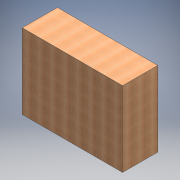
# Autodesk Inventor part: Robot Volume and wall
Saved by Autodesk Inventor 2016 (Build 200138000, 138)
## iProperties
Created: 2017-12-21
Part Number: Robot Volume and wall
Material: Wood (Birch)
Document SubType Name: Modeling
Designer: kornbot
Density: 0.55 g/cm^3
Appearance: Birch - Natural Polished
Author: kornbot
Autodesk Inventor part; units mm, degrees
ref_plane "YZ Plane" through (0, 0, 0) normal (1, 0, 0) x (0, 1, 0)
ref_plane "XZ Plane" through (0, 0, 0) normal (0, 1, 0) x (-1, 0, 0)
ref_plane "XY Plane" through (0, 0, 0) normal (0, 0, 1) x (1, 0, 0)
sketch "Sketch1" plane through (0, 0, 0) normal (0, 0, 1) x (1, 0, 0)
  line L0 (0, 0) -> (0, 700)
  line L1 (0, 0) -> (2000, 0)
  line L2 (0, 700) -> (2000, 700)
  line L3 (2000, 700) -> (2000, 0)
  line L4 (2000, 0) -> (0, 0)
  line L5 (0, 0) -> (0, 700)
  dimension "d0" = 700
  dimension "d1" = 2000
  constraints: 12 end point, 2 horizontal, 2 parallel, 1 perpendicular, 1 vertical
  measures "d0" distance of L0.start L0.end
  measures "d1" distance of L0.start L1.end
extrude "Extrusion1" add sketch "Sketch1" along normal blind 1500
sketch "Sketch2" plane through (0, 700, 0) normal (0, 1, 0) x (1, 0, 0)
  line L0 (1974.1538, -1477.007) -> (20.8481, -1477.007)
  line L1 (20.8481, -1477.007) -> (20.8481, -20.8481)
  line L2 (20.8481, -20.8481) -> (1974.1538, -20.8481)
  line L3 (1974.1538, -20.8481) -> (1974.1538, -1477.007)
  point P0 (0, 0)
  constraints: 8 end point, 2 parallel, 1 horizontal, 1 perpendicular
extrude "Extrusion2" cut sketch "Sketch2" against normal blind 692.25
sketch "Sketch3" plane through (0, 7.75, 0) normal (0, 1, 0) x (1, 0, 0)
  line L0 (1974.1538, -20.8481) -> (1974.1538, -1477.007) projected
  line L1 (20.8481, -20.8481) -> (1974.1538, -20.8481) projected
  line L2 (1974.1538, -1477.007) -> (20.8481, -20.8481)
  line L3 (1974.1538, -1477.007) -> (20.8481, -1477.007) projected
  line L4 (20.8481, -1477.007) -> (1974.1538, -20.8481)
  line L5 (997.5009, -748.9276) -> (997.5009, -1112.664)
  circle A0 centre (997.5009, -1112.664) radius 140.4471
  line L6 (997.5009, -1253.1111) -> (997.5009, -1303.1111)
  circle A1 centre (997.5009, -1303.1111) radius 25
  circle A2 centre (832.5689, -1207.8876) radius 25
  circle A3 centre (832.5689, -1017.4404) radius 25
  circle A4 centre (997.5009, -922.2169) radius 25
  circle A5 centre (1162.433, -1017.4404) radius 25
  circle A6 centre (1162.433, -1207.8876) radius 25
  circle A7 centre (997.5009, -1112.664) radius 226.7645
  circle A8 centre (997.5009, -1112.664) radius 226.7645
  point P0 (0, 0)
  dimension "d9" = 50
  dimension "d11" = 50
  dimension "d14" = 360
  constraints: 8 centre point, 8 end point, 4 coincident, 2 midpoint, 2 vertical, 1 concentric, 1 vertical alignment, 15 other
  measures "d9" distance of L6.start L6.end
  measures "d11" diameter of A1
extrude "Extrusion3" add sketch "Sketch3" along normal blind 112.25 contours A7
body "Solid1"
